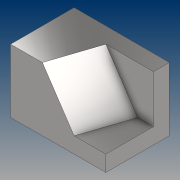
# Autodesk Inventor part: 49
Saved by Autodesk Inventor 2020.2 (Build 242310000, 310)
## iProperties
Created: 2020-09-17
Part Number: 49
Material: 鋼、碳鋼
Document SubType Name: Modeling
Designer: user
Density: 7.85 g/cm^3
Appearance: 半拋光
Mass: 576.975 g
Surface Area: 121.225 cm^2
Volume: 73.5 cm^3
Author: user
Autodesk Inventor part; units mm, degrees
ref_plane "YZ Plane" through (0, 0, 0) normal (1, 0, 0) x (0, 1, 0)
ref_plane "XZ Plane" through (0, 0, 0) normal (0, 1, 0) x (-1, 0, 0)
ref_plane "XY Plane" through (0, 0, 0) normal (0, 0, 1) x (1, 0, 0)
sketch "草圖1" plane through (0, 0, 0) normal (0, 1, 0) x (-1, 0, 0)
  line L0 (0, 0) -> (-60, 0)
  line L1 (-60, 0) -> (-60, 40)
  line L2 (-60, 40) -> (0, 40)
  line L3 (0, 40) -> (0, 0)
  dimension "d0" = 60
  dimension "d1" = 40
  constraints: 8 end point, 2 parallel, 1 horizontal, 1 perpendicular
  measures "d0" distance of L1.end L2.end
  measures "d1" distance of L2.end L0.start
extrude "擠出1" add sketch "草圖1" along normal blind 40
sketch "草圖4" plane through (0, 40, 0) normal (0, 1, 0) x (1, 0, 0)
  line L0 (0, 0) -> (60, 0) projected
  line L1 (60, 0) -> (60, -40) projected
  line L2 (60, -40) -> (0, -40) projected
  line L3 (0, -40) -> (0, 0) projected
  line L4 (0, -40) -> (60, -40) projected
  line L5 (40, -40) -> (50, -10)
  line L6 (50, -10) -> (60, -10)
  dimension "d14" = 10
  dimension "d15" = 10
  dimension "d16" = 20
  constraints: 4 end point, 2 point on line, 1 perpendicular
  measures "d14" distance between parallel lines of L0 L6
  measures "d15" distance of L5.end L6.end
  measures "d16" distance from line of L1 L5.start
extrude "擠出2" cut sketch "草圖4" against normal blind 30 contours L1 L2 L5 L6
sketch "草圖5" plane through (50, 40, 10) normal (0, 0, 1) x (1, 0, 0)
  line L0 (0, 0) -> (0, -30) construction
  line L1 (0, -30) -> (10, -30) projected
  line L2 (10, 0) -> (10, -30) projected
  line L3 (0, 0) -> (10, 0) projected
  line L4 (-50, 0) -> (0, 0) construction
  line L5 (-50, -40) -> (-50, 0) construction
  line L6 (10, -40) -> (-50, -40) construction
  line L7 (10, -30) -> (10, -40) construction
  line L8 (10, -30) -> (0, -30)
  line L9 (0, -30) -> (-20, 0)
  line L10 (10, 0) -> (-50, 0) construction
  line L11 (-20, 0) -> (10, 0)
  line L12 (10, 0) -> (10, -30)
  dimension "d19" = 30
  constraints: 8 end point, 2 collinear, 1 midpoint, 1 perpendicular
  measures "d19" distance from line of L2 L9.end
sketch "草圖6" plane through (0, 10, 0) normal (0, 1, 0) x (1, 0, 0)
  line L0 (50, -10) -> (40, -40) construction
  line L1 (60, -40) -> (40, -40) construction
  line L2 (60, -10) -> (60, -40) construction
  line L3 (60, 0) -> (60, -10) construction
  line L4 (0, 0) -> (60, 0) construction
  line L5 (0, -40) -> (0, 0) construction
  line L6 (40, -40) -> (0, -40) construction
  line L7 (60, -10) -> (50, -10) construction
  line L8 (40, -40) -> (50, -10) projected
  line L9 (50, -10) -> (40, -40)
  constraints: 2 end point, 1 collinear
sweep "掃掠1" cut profiles "草圖5" path "草圖6" path curves L9
